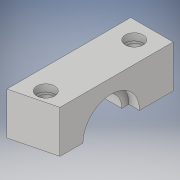
# Autodesk Inventor part: ExtruderClamp
Saved by Autodesk Inventor 2019 (Build 230136000, 136)
## iProperties
Created: 2018-06-27
Part Number: ExtruderClamp
Material: Ogólny
Document SubType Name: Modeling
Designer: Kamil
Density: 1 g/cm^3
Appearance: Domyślna
Author: Kamil
Autodesk Inventor part; units mm, degrees
ref_plane "YZ Plane" through (0, 0, 0) normal (1, 0, 0) x (0, 1, 0)
ref_plane "XZ Plane" through (0, 0, 0) normal (0, 1, 0) x (-1, 0, 0)
ref_plane "XY Plane" through (0, 0, 0) normal (0, 0, 1) x (1, 0, 0)
sketch "Szkic1" plane through (0, 0, 0) normal (0, 1, 0) x (-1, 0, 0)
  line L0 (-6, -17.5) -> (6, -17.5)
  line L1 (6, -17.5) -> (6, 17.5)
  line L2 (6, 17.5) -> (-6, 17.5)
  line L3 (-6, 17.5) -> (-6, -17.5)
  line L4 (-6, -17.5) -> (6, 17.5) construction
  line L5 (6, -17.5) -> (-6, 17.5) construction
  circle A0 centre (0, 12.5) radius 1.75
  circle A1 centre (0, -12.5) radius 1.75
  point P0 (0, 0)
  dimension "d0" = 12
  dimension "d1" = 35
  dimension "d2" = 3.5
  dimension "d3" = 3.5
  constraints: 12 end point, 2 centre point, 2 midpoint, 2 parallel, 1 horizontal, 1 perpendicular
  measures "d0" distance of L2.end L1.end
  measures "d1" distance of L1.end L0.end
  measures "d2" diameter of A0
  measures "d3" diameter of A1
extrude "Wyciągnięcie proste1" add sketch "Szkic1" along normal blind 12
sketch "Szkic2" plane through (6, 0, 17.5) normal (1, 0, 0) x (0, 0, -1)
  arc A0 (25.5, 0) -> (9.5, 0) centre (17.5, 0) ccw
  line L0 (9.5, 0) -> (11.5, 0)
  line L1 (23.5, 0) -> (25.5, 0)
  arc A1 (23.5, 0) -> (11.5, 0) centre (17.5, 0) ccw
  dimension "d7" = 16
  constraints: 4 end point, 4 point on circle, 2 centre point, 2 coincident, 2 point on line, 1 horizontal
  measures "d7" diameter of A0
extrude "Wyciągnięcie proste2" cut sketch "Szkic2" against normal blind 3
sketch "Szkic3" plane through (6, 0, 6) normal (1, 0, 0) x (0, 0, -1)
  line L0 (0, 0) -> (12, 0)
  arc A0 (12, 0) -> (0, 0) centre (6, 0) ccw
  constraints: 2 end point, 2 point on circle, 1 centre point, 1 coincident, 1 horizontal
extrude "Wyciągnięcie proste3" cut sketch "Szkic3" against normal blind 9
sketch "Szkic4" plane through (-6, 0, -17.5) normal (-1, 0, 0) x (0, 0, 1)
  arc A0 (25.5, 0) -> (9.5, 0) centre (17.5, 0) ccw
  line L0 (25.5, 0) -> (9.5, 0)
  dimension "d13" = 16
  constraints: 2 end point, 2 point on circle, 1 centre point, 1 coincident, 1 horizontal
  measures "d13" diameter of A0
sketch "Szkic5" plane through (-6, 0, -17.5) normal (-1, 0, 0) x (0, 0, 1)
  point P0 (17.5, 0)
extrude "Wyciągnięcie proste4" cut sketch "Szkic4" against normal blind 3
sketch "Szkic6" plane through (0, 12, 0) normal (0, 1, 0) x (1, 0, 0)
  circle A0 centre (0, -12.5) radius 2.5
  circle A1 centre (0, 12.5) radius 2.5
  point P0 (0, 0)
  dimension "d16" = 5
  dimension "d17" = 5
  constraints: 2 centre point
  measures "d16" diameter of A0
  measures "d17" diameter of A1
extrude "Wyciągnięcie proste5" cut sketch "Szkic6" against normal blind 2
chamfer "Faza1" distance 12 distance2 3 1 edges at (6, 6, 17.5) measured on face at (-2, 4, 17.5)
